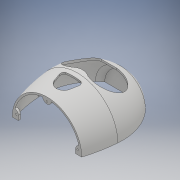
# Autodesk Inventor part: learnbotFront
Saved by Autodesk Inventor 2017 (Build 210142000, 142)
## iProperties
Part Number: learnbotFront
Material: Genérico
Document SubType Name: Modeling
Designer: rober
Density: 1 g/cm^3
Appearance: Valor por defecto
Author: rober
Autodesk Inventor part; units mm, degrees
ref_plane "YZ Plane" through (0, 0, 0) normal (1, 0, 0) x (0, 1, 0)
ref_plane "XZ Plane" through (0, 0, 0) normal (0, 1, 0) x (-1, 0, 0)
ref_plane "XY Plane" through (0, 0, 0) normal (0, 0, 1) x (1, 0, 0)
sketch "Boceto1" plane through (0, 0, 0) normal (0, 0, 1) x (1, 0, 0)
  arc A0 (-1.3629, 5.5333) -> (-0.3139, 0) centre (24.2256, 7.518) ccw
  arc A1 (-1.0638, 5.5565) -> (0, 0) centre (24.2256, 7.518) ccw
  arc A2 (3.3612, 14.9282) -> (1.4714, 13.4053) centre (8.9925, 6.0064) ccw
  arc A3 (3.5214, 14.6745) -> (1.6853, 13.1949) centre (8.9925, 6.0064) ccw
  arc A4 (6.03, 15.7) -> (3.3612, 14.9282) centre (6.03, 10.7) ccw
  arc A5 (6.03, 15.4) -> (3.5214, 14.6745) centre (6.03, 10.7) ccw
  arc A6 (1.4714, 13.4053) -> (-1.3629, 5.5333) centre (8.6002, 6.3924) ccw
  arc A7 (1.6853, 13.1949) -> (-1.0617, 5.5333) centre (8.6002, 6.3924) ccw
  line L0 (6.03, 15.4) -> (6.03, 15.7)
  line L1 (-0.3139, 0) -> (0, 0)
  line L2 (0, 0) -> (-0.3139, 0)
  line L3 (-1.0617, 5.5333) -> (-1.3629, 5.5333)
  arc A8 (-1.0617, 5.5333) -> (0, 0) centre (24.2008, 7.5121) ccw
  arc A9 (-1.3629, 5.5333) -> (-0.3139, 0) centre (24.2256, 7.518) ccw
  line L4 (6.03, 15.7) -> (6.03, 15.4)
  line L5 (4.6409, 15.5032) -> (4.7243, 15.215)
  arc A10 (6.03, 15.7) -> (4.6409, 15.5032) centre (6.03, 10.7) ccw
  arc A11 (6.03, 15.4) -> (4.7243, 15.215) centre (6.03, 10.7) ccw
  point P0 (0, 0)
  constraints: 26 point on circle, 12 centre point, 12 end point, 3 concentric, 1 collinear, 1 horizontal, 1 vertical
revolve "Revolución1" add sketch "Boceto1" angle 180 about axis through (6.03, 15.4, 0) along (0, 1, 0)
sketch "Boceto2" plane through (6.03, 0, 0) normal (0, -1, 0) x (1, 0, 0)
  arc A0 (6.03, 0) -> (-6.03, 0) centre (0, 0) ccw projected
  arc A1 (6.3439, 0) -> (-6.3439, 0) centre (0, 0) ccw projected
  arc A2 (-0.7534, 6.299) -> (0.7534, 6.299) centre (0, 6.03) ccw
  line L0 (0.7534, 6.299) -> (-0.7534, 6.299)
  line L1 (5.23, 0.8) -> (5.23, 0)
  line L2 (5.23, 0) -> (6.03, 0)
  line L3 (7.1298, 0) -> (4.3447, 0) projected
  line L4 (6.03, 0) -> (6.3439, 0)
  line L5 (6.3439, 0) -> (6.1408, 1.5923)
  arc A3 (6.1408, 1.5923) -> (5.23, 0.8) centre (6.03, 0.8) ccw
  arc A4 (6.3362, 0.0609) -> (6.3436, 0.064) centre (6.03, 0.8) ccw
  line L6 (6.3439, 0) -> (5.23, 0)
  line L7 (-5.23, 0.8) -> (-5.23, 0)
  line L8 (-5.23, 0) -> (-6.03, 0)
  line L9 (-7.1298, 0) -> (-4.3447, 0)
  line L10 (-6.3439, 0) -> (-6.1408, 1.5923)
  arc A5 (-5.23, 0.8) -> (-6.1408, 1.5923) centre (-6.03, 0.8) ccw
  line L11 (-6.3439, 0) -> (-5.23, 0)
  point P0 (7.0917, 0)
  dimension "d1" = 1.6
  constraints: 22 end point, 14 point on circle, 4 centre point, 3 collinear, 2 tangent, 1 horizontal, 1 point on line, 1 vertical
  measures "d1" diameter of A2
extrude "Extrusión1" add sketch "Boceto2" against normal blind 0.4 contours L2 L1 A3 A0 | A0 A3 L5 L3 | A2 A0 | A0 A2 L0 | A1 A4 L5 | A5 L7 L8 A0 | A0 L9 L10 A5 picked at (6.2422, 0.914)
sketch "Boceto4" plane through (6.03, 0, 0) normal (0, -1, 0) x (1, 0, 0)
  circle A0 centre (-0.0005, 5.6024) radius 0.15
  circle A1 centre (-5.6181, 0.8021) radius 0.15
  circle A2 centre (5.6033, 0.7979) radius 0.15
  arc A3 (-5.23, 0.8) -> (-5.8214, 1.5723) centre (-6.03, 0.8) ccw projected
  point P0 (-0.8, 0.7979)
  constraints: 3 centre point
extrude "Extrusión2" cut sketch "Boceto4" against normal blind 0.8
sketch "Boceto5" plane through (6.03, 10.7, 0) normal (0, 0, -1) x (-1, 0, 0)
  arc A0 (2.5086, 3.9745) -> (-2.5086, 3.9745) centre (0, 0) ccw
  arc A1 (4.3447, 2.4949) -> (2.5086, 3.9745) centre (-2.9625, -4.6936) ccw
  line L0 (0, 4.7) -> (0, 3.3)
  line L1 (0, 3.3) -> (3.454, 3.3)
  arc A2 (2.5086, 3.9745) -> (0, 4.7) centre (0, 0) ccw
  arc A3 (3.454, 3.3) -> (2.5086, 3.9745) centre (-2.9625, -4.6936) ccw
  point P0 (6.03, -10.7)
  dimension "d10" = 1.4
  constraints: 9 point on circle, 4 centre point, 4 end point, 2 concentric, 1 perpendicular, 1 vertical
  measures "d10" distance of L0.start L0.end
revolve "Revolución2" add sketch "Boceto5" angle 180 about axis through (6.03, 15.4, 0) along (0, 1, 0)
sketch "Boceto6" plane through (6.03, 10.7, 0) normal (0, 0, -1) x (-1, 0, 0)
  line L0 (-1.16, 3.74) -> (-0.44, 3.74)
  line L1 (-0.44, 3.74) -> (-0.44, 4.46)
  line L2 (-0.44, 4.46) -> (-1.16, 4.46)
  line L3 (-1.16, 4.46) -> (-1.16, 3.74)
  line L4 (0.44, 4.46) -> (0.44, 3.74)
  line L5 (0.44, 3.74) -> (1.16, 3.74)
  line L6 (1.16, 3.74) -> (1.16, 4.46)
  line L7 (1.16, 4.46) -> (0.44, 4.46)
  point P0 (6.03, -10.7)
  constraints: 16 end point, 1 perpendicular
extrude "Extrusión3" add sketch "Boceto6" along normal blind 0.4
sketch "Boceto7" plane through (6.03, 10.7, 0) normal (0, 0, -1) x (-1, 0, 0)
  line L0 (-6.25, -10.7) -> (0, -10.7)
  line L1 (6.25, -10.7) -> (0, -10.7)
  arc A0 (1.3838, -4.6009) -> (-1.3837, -4.6009) centre (0, -7.2127) ccw
  arc A1 (-1.3837, 0.5749) -> (1.3838, 0.5749) centre (0, 3.1867) ccw
  arc A2 (0.9515, -4.4143) -> (0.9515, 0.3883) centre (2.2444, -2.013) ccw
  arc A3 (-0.9515, 0.3883) -> (-0.9515, -4.4143) centre (-2.2444, -2.013) ccw
  line L2 (-6.3439, -10.7) -> (-5.23, -10.7) projected
  line L3 (6.3439, -10.7) -> (5.23, -10.7) projected
  arc A4 (-7.3929, -5.1667) -> (-6.3439, -10.7) centre (18.1956, -3.182) ccw projected
  line L4 (6.3439, -10.7) -> (-6.3439, -10.7) projected
  line L5 (-6.3439, -10.7) -> (6.3439, -10.7)
  line L6 (0, -10.7) -> (0, -4.0094)
  point P0 (6.03, -10.7)
  constraints: 16 point on circle, 8 end point, 4 centre point, 1 horizontal, 1 midpoint, 1 vertical
extrude "Extrusión4" cut sketch "Boceto7" against normal blind 40 contours A0 A3 A1 A2
sketch "Boceto8" plane through (6.03, 10.7, 0) normal (0, 0, -1) x (-1, 0, 0)
  line L0 (-6.25, -10.7) -> (0, -10.7)
  line L1 (6.25, -10.7) -> (0, -10.7)
  arc A0 (0, -8.9739) -> (1.44, -7.8939) centre (0.0027, -7.4775) ccw
  arc A1 (-1.44, -7.8939) -> (0, -8.9739) centre (0, -7.4739) ccw
  line L2 (1.3333, -5.9739) -> (-1.3333, -5.9739)
  arc A2 (-1.3333, -5.9739) -> (-1.8133, -6.6139) centre (-1.3333, -6.4739) ccw
  line L3 (-1.8133, -6.6139) -> (-1.44, -7.8939)
  line L4 (1.8133, -6.6139) -> (1.44, -7.8939)
  arc A3 (1.8133, -6.6139) -> (1.3333, -5.9739) centre (1.3333, -6.4739) ccw
  line L5 (-0.7982, -10.7) -> (0.7982, -10.7) projected
  line L6 (0, -10.7) -> (0, -12.145)
  point P0 (6.03, -10.7)
  constraints: 12 end point, 8 point on circle, 4 centre point, 1 midpoint, 1 vertical
extrude "Extrusión5" cut sketch "Boceto8" against normal blind 10
